y_motor_holder (Autodesk Fusion 360 design; units mm, degrees)
Autodesk Fusion 360 part; units mm, degrees
note: some values were not read from the file. Set by a fixed rule: which sketch regions a step uses.
sketch "Sketch1" plane through (0, 0, 0) normal (0, 1, 0) x (1, 0, 0)
  line L0 (0, 0) -> (42.3, 0)
  line L1 (42.3, 0) -> (42.3, -15)
  line L2 (0, 0) -> (0, -42.3)
  line L3 (0, -42.3) -> (15, -42.3)
  circle A0 centre (5.65, -36.65) radius 1.6
  circle A1 centre (5.65, -5.65) radius 1.6
  circle A2 centre (36.65, -5.65) radius 1.6
  line L4 (15, -42.3) -> (15, -30.8674)
  line L5 (42.3, -15) -> (30.8674, -15)
  line L6 (5.65, -36.65) -> (36.65, -5.65) construction
  arc A3 (30.8674, -15) -> (15, -30.8674) centre (21.15, -21.15) ccw
  dimension "d1" = 23
  dimension "d2" = 3.2
  dimension "d3" = 31
  dimension "d4" = 42.3
  dimension "d5" = 42.3
  dimension "d6" = 5.65
  dimension "d7" = 5.65
  dimension "d8" = 31
  dimension "d9" = 15
  dimension "d10" = 15
  constraint coincident L0.start L2.start
  constraint horizontal L0
  constraint perpendicular L0 L1
  constraint perpendicular L0 L2
  constraint perpendicular L2 L3
  constraint equal A1 A2
  constraint equal A0 A1
  constraint vertical A0.centre A1.centre
  constraint horizontal A1.centre A2.centre
  constraint perpendicular L3 L4
  constraint perpendicular L4 L5
  constraint coincident A0.centre L6.start
  constraint coincident A2.centre L6.end
  constraint midpoint A3.centre L6
  measures "d1" diameter of A3
  measures "d2" diameter of A0
  measures "d3" distance of A0.centre A1.centre
  measures "d4" distance of L0 L3
  measures "d5" distance of L0.start L0.end
  measures "d6" distance of L0 A1.centre
  measures "d7" distance of L2 A1.centre
  measures "d8" distance of A1.centre A2.centre
  measures "d9" distance of L2.end L3.end
  measures "d10" distance of L0.end L1.end
extrude "Extrude1" add sketch "Sketch1" along normal blind 4
sketch "Sketch2" plane through (0, 0, 0) normal (-1, 0, 0) x (0, -1, 0)
  line L0 (0, 0) -> (0, 42.3)
  line L1 (0, 42.3) -> (-4, 42.3)
  line L2 (-4, 42.3) -> (-4, 0)
  line L3 (-4, 0) -> (0, 0)
  line L4 (-12, 0) -> (24, 0)
  line L5 (24, 0) -> (24, 30)
  line L6 (24, 30) -> (-12, 30)
  line L7 (-12, 30) -> (-12, 0)
  circle A0 centre (-8, 15) radius 1.6
  circle A1 centre (20, 15) radius 1.6
  dimension "d13" = 3.2
  dimension "d14" = 3.2
  dimension "d15" = 4
  dimension "d16" = 4
  dimension "d17" = 30
  dimension "d18" = 15
  dimension "d19" = 20
  dimension "d20" = 4
  constraint horizontal L4
  constraint vertical L5
  constraint horizontal L6
  constraint vertical L7
  constraint collinear L3 L4
  constraint horizontal A0.centre A1.centre
  measures "d13" diameter of A0
  measures "d14" diameter of A1
  measures "d15" distance of L2 A0.centre
  measures "d16" distance of L7 A0.centre
  measures "d17" distance of L4.start L6.end
  measures "d18" distance of L4 A0.centre
  measures "d19" distance of L0 A1.centre
  measures "d20" distance of L5 A1.centre
extrude "Extrude2" add sketch "Sketch2" along normal blind 5
sketch "Sketch3" plane through (0, 0, 0) normal (1, 0, 0) x (0, 1, 0)
  line L0 (0, 0) -> (0, 30)
  line L1 (0, 30) -> (-24, 30)
  line L2 (-24, 30) -> (-24, 0)
  line L3 (-24, 0) -> (0, 0)
  circle A0 centre (-20, 15) radius 1.6
  circle A1 centre (-20, 15) radius 3.25
  circle A2 centre (8, 15) radius 1.6
  circle A3 centre (8, 15) radius 3.25
  dimension "d23" = 6.5
  constraint concentric A0 A1
  constraint concentric A2 A3
  constraint equal A1 A3
  measures "d23" diameter of A1
extrude "Extrude3" cut sketch "Sketch3" against normal blind 3.5 contours A1
chamfer "Chamfer1" distance 5 angle 45 2 edges at (0, 4, 15) (-2.5, 4, 30)
fillet "Fillet1" radius 3 9 edges at (-2.5, -24, 30) (-2.5, -24, 0) (-2.5, 12, 0) (-2.5, 12, 30) (15, 2, 30.8674) (30.8674, 2, 15) (42.3, 2, 15) (42.3, 2, 0) (15, 2, 42.3)
extrude "Extrude4" cut sketch "Sketch3" along normal through all contours A3
sketch "Sketch4" plane through (0, 4, 0) normal (0, 1, 0) x (-1, 0, 0)
  arc A0 (-12, 42.3) -> (-15, 39.3) centre (-12, 39.3) ccw
  line L0 (-15, 39.3) -> (-15, 32.3984)
  arc A1 (-15, 32.3984) -> (-13.8931, 30.0712) centre (-12, 32.3984) ccw
  arc A2 (-30.0712, 13.8931) -> (-13.8931, 30.0712) centre (-21.15, 21.15) ccw
  arc A3 (-30.0712, 13.8931) -> (-32.3984, 15) centre (-32.3984, 12) ccw
  line L1 (-32.3984, 15) -> (-39.3, 15)
  arc A4 (-39.3, 15) -> (-42.3, 12) centre (-39.3, 12) ccw
  line L2 (-42.3, 12) -> (-42.3, 3)
  arc A5 (-42.3, 3) -> (-39.3, 0) centre (-39.3, 3) ccw
  line L3 (-39.3, 0) -> (-5, 0)
  line L4 (-5, 0) -> (-5, 4.188)
  arc A6 (-5, 7.112) -> (-5, 4.188) centre (-5.65, 5.65) ccw
  line L5 (-5, 7.112) -> (-5, 35)
  line L6 (-5, 35) -> (5, 35)
  line L7 (5, 35) -> (5, 42.3)
  line L8 (5, 42.3) -> (-12, 42.3)
  circle A7 centre (-36.65, 5.65) radius 1.6
  circle A8 centre (-5.65, 36.65) radius 1.6
  circle A9 centre (-5.65, 36.65) radius 3.25
  circle A10 centre (-5.65, 5.65) radius 3.25
  dimension "d30" = 6.5
  constraint concentric A8 A9
  constraint concentric A6 A10
  constraint equal A9 A10
  measures "d30" diameter of A9
extrude "Extrude5" cut sketch "Sketch4" along normal through all contours L5 L6 A9 | L5 L6 A9 | L4 A6 L5 A10 | L4 A6 L5 A10
equation "d5 = d4"
equation "d6 = ( ( 42.3 - 31 ) / 2 ) * 1 mm"
equation "d7 = d6"
equation "d8 = d3"
equation "d10 = d9"
equation "d16 = d15"
equation "d18 = d17 / 2"
equation "d20 = d15"
